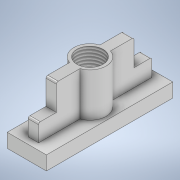
# Autodesk Inventor part: fixação do pino
Saved by Autodesk Inventor 2022 (Build 260153000, 153)
## iProperties
Created: 2023-07-19
Part Number: fixação do pino
Material: Aluminum 6061-AHC
Document SubType Name: Modeling
Designer: Usuário
Density: 2.7 g/cm^3
Appearance: Aluminum - Dark
Author: Usuário
Autodesk Inventor part; units mm, degrees
ref_plane "YZ Plane" through (0, 0, 0) normal (1, 0, 0) x (0, 1, 0)
ref_plane "XZ Plane" through (0, 0, 0) normal (0, 1, 0) x (-1, 0, 0)
ref_plane "XY Plane" through (0, 0, 0) normal (0, 0, 1) x (1, 0, 0)
sketch "Sketch1" plane through (0, 0, 0) normal (0, 1, 0) x (-1, 0, 0)
  line L0 (0, 0) -> (-4.5, 0)
  line L1 (-4.5, 0) -> (-4.5, -14.5)
  line L2 (-4.5, -14.5) -> (0, -14.5)
  line L3 (0, -14.5) -> (0, 0)
  circle A0 centre (-2.25, -7.25) radius 1.5
  line L4 (-1.65, -13.75) -> (-1.65, -9)
  line L5 (-1.65, -5.5) -> (-1.65, -0.75)
  line L6 (-2.85, -13.75) -> (-2.85, -9)
  line L7 (-2.85, -5.5) -> (-2.85, -0.75)
  line L8 (-1.65, -0.75) -> (-2.85, -0.75)
  line L9 (-1.65, -13.75) -> (-2.85, -13.75)
  line L10 (-1.65, -11.7) -> (-2.85, -11.7)
  line L11 (-1.65, -2.8) -> (-2.85, -2.8)
  circle A1 centre (-2.25, -7.25) radius 1.85
  dimension "d0" = 4.5
  dimension "d2" = 3
  dimension "d9" = 3.7
  dimension "d32" = 7.25
  dimension "d33" = 7.25
  constraints: 24 end point, 4 point on circle, 4 point on line, 3 horizontal, 2 centre point, 2 parallel, 1 coincident, 1 perpendicular
  measures "d0" distance of L2.end L1.end
  measures "d2" diameter of A0
  measures "d9" diameter of A1
  measures "d32" distance from line of A0.centre L2
  measures "d33" distance from line of L0 A0.centre
extrude "Extrusion1" add sketch "Sketch1" against normal blind 1.6 contours L3 L2 L1 L0 | A0 | L9 L6 L10 L4 | L10 L6 A1 L4 | A1 | L7 L11 L5 A1 | L7 L8 L5 L11
extrude "Extrusion2" add sketch "Sketch1" along normal blind 2 contours L9 L6 L10 L4 | L7 L8 L5 L11
extrude "Extrusion3" add sketch "Sketch1" along normal blind 5 contours L10 L6 A1 L4 | A1 | L7 L11 L5 A1
fillet "Fillet1" radius 0.2 4 edges at (2.25, 5, -2.8) (2.25, 5, -11.7) (2.25, 2, -0.75) (2.25, 2, -13.75)
thread "Thread1" size "M3x0.35" class "6H" standard "ANSI Metric M Profile" length 8.5
sketch "Sketch2" plane through (2.25, 0, -7.25) normal (0, 1, 0) x (1, 0, 0)
  circle A0 centre (0, 0) radius 1.5 projected
  point P0 (-2.25, -7.25)
extrude "Extrusion4" cut sketch "Sketch2" against normal blind 10
body "Solid1"
